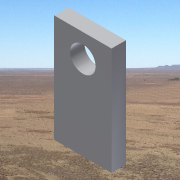
# Autodesk Inventor part: 2f1ah
Saved by Autodesk Inventor 2014 SP1 (Build 180222100, 222)
## iProperties
Company: HERA Project
Created: 2013-12-20
Part Number: 2f1ah
Material: PBT Plastic
Description: Arm holder
Document SubType Name: Modeling
Designer: Rich Bradley
Mass: 70.9499 g
Surface Area: 134.863 cm^2
Volume: 56.3542 cm^3
Density: 1.259 g/cm^3
Appearance: Smooth - White
Title: Dipole arm holder
Author: Dave
Autodesk Inventor part; units mm, degrees
ref_plane "YZ Plane" through (0, 0, 0) normal (1, 0, 0) x (0, 1, 0)
ref_plane "XZ Plane" through (0, 0, 0) normal (0, 1, 0) x (-1, 0, 0)
ref_plane "XY Plane" through (0, 0, 0) normal (0, 0, 1) x (1, 0, 0)
sketch "Sketch1" plane through (0, 0, 0) normal (0, 0, 1) x (1, 0, 0)
  line L0 (0, 0) -> (50.8, 0)
  line L1 (50.8, 0) -> (50.8, 95.25)
  line L2 (50.8, 95.25) -> (0, 95.25)
  line L3 (0, 95.25) -> (0, 0)
  dimension "d0" = 50.8
  dimension "d1" = 95.25
  constraints: 8 end point, 2 parallel, 1 horizontal, 1 perpendicular
  measures "d0" distance of L0.start L0.end
  measures "d1" distance of L2.end L0.start
extrude "Extrusion1" add sketch "Sketch1" along normal blind 12.7
sketch "Sketch2" plane through (0, 0, 12.7) normal (0, 0, 1) x (1, 0, 0)
  line L0 (0, 0) -> (50.8, 0) projected
  circle A0 centre (25.4, 74.549) radius 11.303
  dimension "d4" = 74.549
  dimension "d5" = 22.606
  constraints: 1 centre point
  measures "d4" distance from line of L0 A0.centre
  measures "d5" diameter of A0
extrude "Extrusion2" cut sketch "Sketch2" against normal blind 12.7
sketch "Sketch3" plane through (0, 0, 0) normal (0, -1, 0) x (1, 0, 0)
  line L0 (0, 0) -> (50.8, 0) projected
  line L1 (0, 12.7) -> (50.8, 12.7) projected
  line L2 (25.4, 12.7) -> (25.4, 0) construction
  circle A0 centre (7.1374, 6.35) radius 2.4611
  circle A1 centre (43.6626, 6.35) radius 2.4611
  dimension "d8" = 18.2626
  constraints: 2 centre point, 2 end point, 2 midpoint, 1 symmetric about line, 1 other
  measures "d8" distance from line of A0.centre L2
hole "Hole1" at (7.1374, 0, 6.35) at (43.6626, 0, 6.35) direction (0, 1, 0) diameter 3.302 depth 15.24 tip angle 118 thread size "8-32 UNC" class "2B" standard "ANSI Unified Screw Threads"
body "Solid1"
